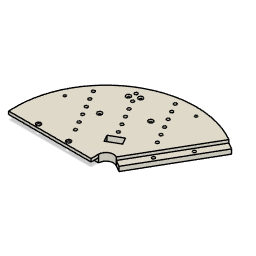
Base (Autodesk Fusion 360 design; units mm, degrees)
Autodesk Fusion 360 part; units mm, degrees
sketch "Sketch1" plane through (0, 0, 0) normal (0, 1, 0) x (1, 0, 0)
  line L0 (-120, 0) -> (-10, 0)
  line L1 (5, 8.6603) -> (60, 103.923)
  arc A0 (60, 103.923) -> (-120, 0) centre (0, 0) ccw
  arc A1 (5, 8.6603) -> (-10, 0) centre (0, 0) ccw
  dimension "d57" = 240
  dimension "d58" = 120
  dimension "d59" = 20
  constraint coincident A0.centre A1.centre
  constraint horizontal L0
  constraint coincident L0 A0.centre
  constraint coincident A0.centre L1
  measures "d57" diameter of A0
  measures "d58" angle of L0 L1
  measures "d59" diameter of A1
extrude "Extrude3" add sketch "Sketch1" along normal blind 10
sketch "Sketch9" plane through (0, 0, 0) normal (0, 0, 1) x (1, 0, 0)
  line L0 (-120, 0) -> (-10, 0)
  line L1 (-10, 0) -> (-10, 10)
  line L2 (-10, 10) -> (-120, 10)
  line L3 (-120, 10) -> (-120, 0)
  line L4 (-120, 10) -> (-10, 10)
  line L5 (-10, 10) -> (-10, 6)
  line L6 (-10, 6) -> (-120, 6)
  line L7 (-120, 6) -> (-120, 10)
  dimension "d60" = 4
  constraint horizontal L4
  constraint vertical L5
  constraint horizontal L6
  constraint vertical L7
  constraint coincident L2.end L3.start
  measures "d60" distance of L2.end L6.end
extrude "Extrude8" add sketch "Sketch9" along normal blind 10 contours L1 L2 L3 L4 L5 L6 L7
sketch "Sketch12" plane through (0, 0, 0) normal (0.866025, 0, 0.5) x (0.5, 0, -0.866025)
  line L0 (10, 0) -> (120, 0)
  line L1 (120, 0) -> (120, 10)
  line L2 (120, 10) -> (10, 10)
  line L3 (10, 10) -> (10, 0)
  line L4 (10, 0) -> (120, 0)
  line L5 (120, 0) -> (120, 6)
  line L6 (120, 6) -> (10, 6)
  line L7 (10, 6) -> (10, 0)
  dimension "d63" = 6
  constraint horizontal L4
  constraint vertical L5
  constraint horizontal L6
  constraint vertical L7
  constraint coincident L0.start L3.end
  measures "d63" distance of L0.start L6.end
extrude "Extrude9" add sketch "Sketch12" along normal blind 10 contours L0 L1 L3 L4 L5 L6 L7
sketch "Sketch13" plane through (0, 10, 0) normal (0, 1, 0) x (-1, 0, 0)
  arc A0 (-60, -103.923) -> (120, 0) centre (0, 0) ccw
  line L0 (120, 0) -> (120, 10)
  line L1 (120, 10) -> (10, 10)
  line L2 (10, 10) -> (10, 0)
  arc A1 (-5, -8.6603) -> (10, 0) centre (0, 0) ccw
  line L3 (-5, -8.6603) -> (-60, -103.923)
  point P0 (85, 5)
  point P1 (45, 5)
  dimension "d68" = 35
  dimension "d69" = 35
  measures "d68" distance of L2 P1
  measures "d69" distance of L0 P0
hole "Hole1" at (-85, 10, 5) at (-45, 10, 5) direction (0, -1, 0) diameter 4 depth 4 tip angle 118 countersink diameter 6 countersink angle 90
sketch "Sketch14" plane through (0, 6, 0) normal (0, 1, 0) x (-1, 0, 0)
  line L0 (-60, -103.923) -> (-5, -8.6603)
  line L1 (-5, -8.6603) -> (-13.6603, -3.6603)
  line L2 (-13.6603, -3.6603) -> (-68.6603, -98.923)
  line L3 (-68.6603, -98.923) -> (-60, -103.923)
  line L4 (-9.3301, -6.1603) -> (-64.3301, -101.423) construction
  point P0 (-26.8301, -36.4711)
  point P1 (-46.8301, -71.1122)
  dimension "d75" = 35
  dimension "d76" = 35
  constraint midpoint L1 L4.start
  constraint midpoint L3 L4.end
  constraint coincident L4 P0
  constraint coincident L4 P1
  measures "d75" distance of L1 P0
  measures "d76" distance of L3 P1
hole "Hole2" at (26.8301, 6, -36.4711) at (46.8301, 6, -71.1122) direction (0, -1, 0) diameter 4 depth 15 tip angle 118
sketch "Sketch15" plane through (0, 10, 0) normal (0, 1, 0) x (-1, 0, 0)
  circle A0 centre (85, 5) radius 3
  circle A1 centre (45, 5) radius 3
  arc A2 (-60, -103.923) -> (120, 0) centre (0, 0) ccw
  line L0 (120, 0) -> (120, 10)
  line L1 (120, 10) -> (10, 10)
  line L2 (10, 10) -> (10, 0)
  arc A3 (-5, -8.6603) -> (10, 0) centre (0, 0) ccw
  line L3 (-5, -8.6603) -> (-60, -103.923)
  line L4 (0, 0) -> (60, -103.923) construction
  line L5 (10, 0) -> (120, 0)
  line L6 (56.6506, -48.1218) -> (13.3494, -73.1218) construction
  line L7 (5.7058, -27.8827) -> (21.2942, -18.8827)
  line L8 (5.7058, -27.8827) -> (10.7058, -36.5429)
  line L9 (10.7058, -36.5429) -> (26.2942, -27.5429)
  line L10 (26.2942, -27.5429) -> (21.2942, -18.8827)
  line L11 (57.1962, -87.0666) -> (46.8038, -93.0666) construction
  dimension "d80" = 60
  dimension "d81" = 50
  dimension "d82" = 25
  dimension "d83" = 50
  dimension "d89" = 43
  dimension "d90" = 9
  dimension "d91" = 18
  dimension "d92" = 10
  dimension "d95" = 6
  dimension "d96" = 12
  dimension "d97" = 34
  constraint coincident A2.centre A3.centre
  constraint coincident A2 L4.end
  constraint perpendicular L4 L6
  constraint perpendicular L4 L7
  constraint perpendicular L7 L8
  constraint perpendicular L8 L9
  constraint perpendicular L7 L10
  constraint perpendicular L4 L11
  measures "d80" angle of L4 L5
  measures "d81" distance of L6.start L6.end
  measures "d82" distance of L4 L6.end
  measures "d83" distance of L4.end L6
  measures "d89" distance of L6 L7
  measures "d90" distance of L4 L7.start
  measures "d91" distance of L7.start L7.end
  measures "d92" distance of L7 L9
  measures "d95" distance of L4 L11.start
  measures "d96" distance of L11.start L11.end
  measures "d97" distance of L6 L11
hole "Hole3" at (-56.6506, 10, -48.1218) at (-13.3494, 10, -73.1218) at (-57.1962, 10, -87.0666) at (-46.8038, 10, -93.0666) direction (0, -1, 0) diameter 3.2 depth 35 tip angle 118 countersink diameter 6 countersink angle 90
extrude "Extrude10" cut sketch "Sketch15" against normal blind 20 contours L7 L8 L9 L10
sketch "Sketch16" plane through (0, 10, 0) normal (0, 1, 0) x (-1, 0, 0)
  line L0 (120, 0) -> (120, 10)
  line L1 (10, 0) -> (10, 10)
  line L2 (-5, -8.6603) -> (-13.6603, -3.6603)
  line L3 (-60, -103.923) -> (-68.6603, -98.923)
  line L4 (120, 5) -> (10, 5) construction
  line L5 (-9.3301, -6.1603) -> (-64.3301, -101.423) construction
  line L6 (-11.0289, -109.1025) -> (-97.6314, -59.1025) construction
  line L7 (100, -45) -> (100, 55) construction
  dimension "d98" = 100
  dimension "d99" = 50
  dimension "d100" = 20
  dimension "d101" = 20
  dimension "d102" = 100
  dimension "d103" = 50
  constraint midpoint L0 L4.start
  constraint midpoint L1 L4.end
  constraint midpoint L2 L5.start
  constraint midpoint L3 L5.end
  constraint vertical L7
  constraint perpendicular L5 L6
  measures "d98" distance of L6.start L6.end
  measures "d99" distance of L5 L6.start
  measures "d100" distance of L3 L6
  measures "d101" distance of L0 L7
  measures "d102" distance of L7.start L7.end
  measures "d103" distance of L4 L7.start
sketch "Sketch17" plane through (0, 0, 0) normal (0, -1, 0) x (1, 0, 0)
  line L0 (-10.7058, -36.5429) -> (-26.2942, -27.5429)
  line L1 (-26.2942, -27.5429) -> (-21.2942, -18.8827)
  line L2 (-21.2942, -18.8827) -> (-5.7058, -27.8827)
  line L3 (-5.7058, -27.8827) -> (-10.7058, -36.5429)
  circle A0 centre (-57.1962, -87.0666) radius 1.6
  circle A1 centre (-56.6506, -48.1218) radius 1.6
  circle A2 centre (-13.3494, -73.1218) radius 1.6
  circle A3 centre (-46.8038, -93.0666) radius 1.6
  circle A4 centre (26.8301, -36.4711) radius 2
  circle A5 centre (46.8301, -71.1122) radius 2
  arc A6 (-120, 0) -> (60, -103.923) centre (0, 0) ccw
  line L4 (60, -103.923) -> (68.6603, -98.923)
  line L5 (68.6603, -98.923) -> (13.6603, -3.6603)
  line L6 (13.6603, -3.6603) -> (5, -8.6603)
  arc A7 (-10, 0) -> (5, -8.6603) centre (0, 0) ccw
  line L7 (-10, 0) -> (-120, 0)
sketch "Sketch18" plane through (0, 0, 0) normal (0, -1, 0) x (1, 0, 0)
  point P0 (-100, -45)
  point P1 (11.0289, -109.1025)
  point P2 (-100, -45)
  point P3 (11.0289, -109.1025)
  constraint coincident P2 P0
  constraint coincident P3 P1
hole "Hole4" at (-100, 0, -45) at (11.0289, 0, -109.1025) direction (0, 1, 0) diameter 3.2 depth 25 tip angle 180 countersink diameter 6 countersink angle 90
sketch "Sketch19" plane through (0, 10, 0) normal (0, 1, 0) x (-1, 0, 0)
  circle A0 centre (100, -45) radius 1.6
  circle A1 centre (-11.0289, -109.1025) radius 1.6
  line L0 (26.2942, -27.5429) -> (10.7058, -36.5429)
  line L1 (10.7058, -36.5429) -> (5.7058, -27.8827)
  line L2 (5.7058, -27.8827) -> (21.2942, -18.8827)
  line L3 (21.2942, -18.8827) -> (26.2942, -27.5429)
  circle A2 centre (57.1962, -87.0666) radius 3
  circle A3 centre (56.6506, -48.1218) radius 3
  circle A4 centre (13.3494, -73.1218) radius 3
  circle A5 centre (46.8038, -93.0666) radius 3
  circle A6 centre (85, 5) radius 3
  circle A7 centre (45, 5) radius 3
  arc A8 (-60, -103.923) -> (120, 0) centre (0, 0) ccw
  line L4 (120, 0) -> (120, 10)
  line L5 (120, 10) -> (10, 10)
  line L6 (10, 10) -> (10, 0)
  arc A9 (-5, -8.6603) -> (10, 0) centre (0, 0) ccw
  line L7 (-5, -8.6603) -> (-60, -103.923)
  line L8 (5, -8.6603) -> (60, -103.923) construction
  line L9 (91.2096, -77.9796) -> (46.188, 0) construction
  line L10 (21.9275, -117.9796) -> (-23.094, -40) construction
  line L11 (10, 0) -> (120, 0)
  circle A10 centre (86.2096, -69.3193) radius 2
  circle A11 centre (16.9275, -109.3193) radius 2
  circle A12 centre (55, -95.2628) radius 2
  point P0 (120, 5)
  dimension "d111" = 40
  dimension "d112" = 40
  dimension "d113" = 4
  dimension "d114" = 10
  dimension "d115" = 4
  dimension "d116" = 10
  dimension "d117" = 4
  dimension "d118" = 10
  constraint midpoint A9 L8.start
  constraint midpoint A8 L8.end
  constraint parallel L8 L10
  constraint parallel L8 L9
  constraint coincident A8 L9.start
  constraint coincident A8 L10.start
  constraint coincident L7 L10.end
  constraint coincident L9.end L11
  constraint coincident L9 A10.centre
  constraint coincident L10 A11.centre
  constraint coincident L8 A12.centre
  measures "d111" distance of L8 L9
  measures "d112" distance of L8 L10
  measures "d113" diameter of A10
  measures "d114" distance of L9.start A10.centre
  measures "d115" diameter of A11
  measures "d116" distance of L10.start A11.centre
  measures "d117" diameter of A12
  measures "d118" distance of L8.end A12.centre
extrude "Extrude11" cut sketch "Sketch19" against normal blind 80 contours A10 | A11 | A12
pattern_linear "R-Pattern1" count 6 spacing 13 along (0.5, 0, 0.866025) of "Extrude11"
equation "d82 = d81 / 2"
equation "d90 = d91 / 2"
equation "d96 = d95 * 2"
equation "d99 = d98 / 2"
equation "d101 = d100"
equation "d102 = d98"
equation "d103 = d99"
equation "d112 = d111"
equation "d116 = d114"
equation "d118 = d114"
